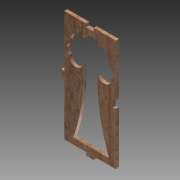
# Autodesk Inventor part: Birdhouse Wall
Saved by Autodesk Inventor 2015 (Build 190159000, 159)
## iProperties
Created: 2018-03-09
Part Number: Birdhouse Wall
Material: Wood (Birch)
Document SubType Name: Modeling
Designer: Administrator
Density: 0.55 g/cm^3
Appearance: Birch - Natural Polished
Mass: 5.89524 g
Surface Area: 88.8018 cm^2
Volume: 10.7186 cm^3
Author: Administrator
Autodesk Inventor part; units mm, degrees
ref_plane "YZ Plane" through (0, 0, 0) normal (1, 0, 0) x (0, 1, 0)
ref_plane "XZ Plane" through (0, 0, 0) normal (0, 1, 0) x (-1, 0, 0)
ref_plane "XY Plane" through (0, 0, 0) normal (0, 0, 1) x (1, 0, 0)
sketch "Sketch1" plane through (0, 0, 0) normal (0, 0, 1) x (1, 0, 0)
  line L0 (0, 0) -> (52.9336, 0)
  line L1 (52.9336, 0) -> (52.9336, 114.3)
  line L2 (52.9336, 114.3) -> (0, 114.3)
  line L3 (0, 114.3) -> (0, 0)
  dimension "d0" = 114.3
  dimension "d1" = 52.9336
  constraints: 8 end point, 2 parallel, 1 horizontal, 1 perpendicular
  measures "d0" distance of L2.end L0.start
  measures "d1" distance of L0.start L0.end
extrude "Extrusion1" add sketch "Sketch1" along normal blind 3.175
sketch "Sketch2" plane through (0, 0, 3.175) normal (0, 0, 1) x (1, 0, 0)
  line L0 (0, 114.3) -> (0, 0) projected
  line L1 (52.9336, 0) -> (52.9336, 114.3) projected
  line L2 (0, 60.96) -> (-3.175, 60.96)
  line L3 (-3.175, 60.96) -> (-3.175, 53.34)
  line L4 (-3.175, 53.34) -> (0, 53.34)
  line L5 (0, 53.34) -> (0, 60.96)
  line L6 (52.9336, 60.96) -> (49.7586, 60.96)
  line L7 (49.7586, 60.96) -> (49.7586, 53.34)
  line L8 (49.7586, 53.34) -> (52.9336, 53.34)
  line L9 (52.9336, 53.34) -> (52.9336, 60.96)
  line L10 (52.9336, 114.3) -> (0, 114.3) projected
  line L11 (0, 0) -> (52.9336, 0) projected
  line L12 (30.2768, 114.3) -> (22.6568, 114.3)
  line L13 (30.2768, 0) -> (30.2768, -3.175)
  line L14 (30.2768, -3.175) -> (22.6568, -3.175)
  line L15 (22.6568, -3.175) -> (22.6568, 0)
  line L16 (22.6568, 0) -> (30.2768, 0)
  line L17 (22.6568, 114.3) -> (22.6568, 111.125)
  line L18 (22.6568, 111.125) -> (30.2768, 111.125)
  line L19 (30.2768, 111.125) -> (30.2768, 114.3)
  point P0 (0, 57.15)
  point P1 (52.9336, 57.15)
  point P2 (26.4668, 114.3)
  point P3 (26.4668, 0)
  dimension "d4" = 3.81
  dimension "d5" = 7.62
  dimension "d6" = 3.175
  dimension "d7" = 3.81
  dimension "d8" = 7.62
  dimension "d9" = 3.175
  dimension "d13" = 7.62
  dimension "d14" = 3.81
  dimension "d15" = 3.175
  dimension "d20" = 7.62
  dimension "d21" = 3.81
  dimension "d22" = 3.175
  constraints: 32 end point, 8 point on line, 7 perpendicular, 6 parallel, 4 midpoint, 2 collinear, 2 vertical
  measures "d4" distance from line of point (0, 57.15) L2
  measures "d5" distance between parallel lines of L2 L4
  measures "d6" distance between parallel lines of L0 L3
  measures "d7" distance from line of point (52.934, 57.15) L6
  measures "d8" distance between parallel lines of L6 L8
  measures "d9" distance between parallel lines of L1 L7
  measures "d13" distance between parallel lines of L13 L15
  measures "d14" distance from line of L13 point (26.467, 0)
  measures "d15" distance between parallel lines of L14 L11
  measures "d20" distance between parallel lines of L17 L19
  measures "d21" distance from line of L19 point (26.467, 114.3)
  measures "d22" distance between parallel lines of L10 L18
extrude "Extrusion2" add sketch "Sketch2" against normal blind 3.175 contours L0 L4 L3 L2 | L10 L19 L18 L17 | L11 L13 L14 L15 | L1 L8 L7 L6
extrude "Extrusion3" cut sketch "Sketch2" against normal blind 3.175 contours L10 L19 L18 L17 | L1 L8 L7 L6
sketch "Sketch3" plane through (0, 0, 3.175) normal (0, 0, 1) x (1, 0, 0)
  line L0 (0, 60.96) -> (0, 114.3)
  line L1 (22.6568, 114.3) -> (0, 114.3) projected
  line L2 (0, 114.3) -> (22.6568, 114.3)
  line L3 (22.6568, 114.3) -> (22.6568, 111.125)
  line L4 (22.6568, 111.125) -> (30.2768, 111.125)
  line L5 (30.2768, 111.125) -> (22.6568, 111.125) projected
  line L6 (30.2768, 111.125) -> (30.2768, 114.3)
  line L7 (30.2768, 114.3) -> (52.9336, 114.3)
  line L8 (52.9336, 114.3) -> (52.9336, 60.96)
  line L9 (52.9336, 60.96) -> (52.9336, 114.3) projected
  line L10 (52.9336, 60.96) -> (49.7586, 60.96)
  line L11 (49.7586, 60.96) -> (49.7586, 53.34)
  line L12 (49.7586, 60.96) -> (49.7586, 53.34) projected
  line L13 (49.7586, 53.34) -> (52.9336, 53.34)
  line L14 (52.9336, 53.34) -> (52.9336, 0)
  line L15 (52.9336, 0) -> (52.9336, 53.34) projected
  line L16 (52.9336, 0) -> (30.2768, 0)
  line L17 (0, 0) -> (22.6568, 0) projected
  line L18 (30.2768, 0) -> (30.2768, -3.175)
  line L19 (30.2768, -3.175) -> (22.6568, -3.175)
  line L20 (22.6568, -3.175) -> (30.2768, -3.175) projected
  line L21 (22.6568, -3.175) -> (22.6568, 0)
  line L22 (22.6568, 0) -> (0, 0)
  line L23 (0, 0) -> (0, 53.34)
  line L24 (0, 53.34) -> (0, 0) projected
  line L25 (0, 53.34) -> (-3.175, 53.34)
  line L26 (-3.175, 53.34) -> (-3.175, 60.96)
  line L27 (-3.175, 60.96) -> (-3.175, 53.34) projected
  line L28 (-3.175, 60.96) -> (0, 60.96)
  constraints: 40 end point, 10 perpendicular, 9 collinear
sketch "Sketch4" plane through (0, 0, 3.175) normal (0, 0, 1) x (1, 0, 0)
  arc A0 (9.4645, 6.35) -> (18.9927, 77.7875) centre (-158.3531, 65.0875) ccw
  arc A1 (34.4743, 77.7875) -> (46.0375, 6.35) centre (212.0985, 69.884) ccw
  line L0 (0, 0) -> (22.6568, 0) projected
  line L1 (30.2768, 0) -> (52.9336, 0) projected
  line L2 (9.4645, 6.35) -> (46.0375, 6.35)
  arc A2 (4.7619, 76.2078) -> (18.9927, 77.7875) centre (11.8465, 77.2757) ccw
  arc A3 (6.7319, 88.6305) -> (4.6889, 77.5927) centre (8.7235, 82.5539) ccw
  arc A4 (4.6889, 77.5927) -> (4.7619, 76.2078) centre (11.8465, 77.2757) ccw
  arc A5 (19.9033, 100.0791) -> (6.7319, 88.6305) centre (15.9469, 91.3299) ccw
  line L3 (26.4922, 114.3) -> (26.4922, 47.625) construction
  line L4 (52.9336, 60.96) -> (52.9336, 114.3) projected
  arc A6 (34.37, 74.925) -> (48.2225, 76.2078) centre (41.1379, 77.2757) ccw
  arc A7 (48.2955, 77.5927) -> (46.2525, 88.6305) centre (44.2609, 82.5539) ccw
  arc A8 (48.2225, 76.2078) -> (48.2955, 77.5927) centre (41.1379, 77.2757) ccw
  arc A9 (46.2525, 88.6305) -> (35.0777, 100.7299) centre (37.0375, 91.3299) ccw
  arc A10 (35.0777, 100.7299) -> (19.9033, 100.0791) centre (27.6731, 96.1477) ccw
  point P0 (21.8385, 98.9122)
  point P1 (33.9917, 77.7875)
  point P2 (31.1459, 98.9122)
  dimension "d23" = 71.4375
  dimension "d24" = 6.35
  dimension "d25" = 177.8
  dimension "d26" = 6.35
  dimension "d28" = 177.8
  dimension "d29" = 26.4414
  dimension "d30" = 71.4375
  constraints: 23 point on circle, 11 centre point, 9 symmetric about line, 4 end point, 1 tangent, 1 vertical, 4 other
  measures "d23" vertical distance of L2.start A0.end
  measures "d24" distance from line of L0 L2.start
  measures "d25" radius of A0
  measures "d26" distance from line of L1 L2.end
  measures "d28" radius of A1
  measures "d29" distance between parallel lines of L4 L3
  measures "d30" vertical distance of A1.start L2.end
extrude "Extrusion4" cut sketch "Sketch4" against normal blind 25.4
body "Solid1"
